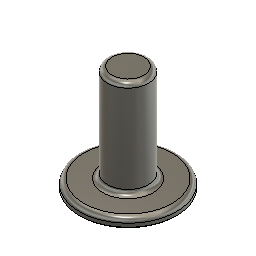
Stick_Topper (Autodesk Fusion 360 archive; units mm, degrees)
design "Stick Topper"
part number: Medium
Autodesk Fusion 360 part; units mm, degrees
sketch "Sketch1" plane through (0, 0, 0) normal (0, 0, 1) x (1, 0, 0)
  line L0 (0, 0) -> (14, 0)
  line L1 (14, 0) -> (14, -6)
  line L2 (14, -6) -> (41.5, -6)
  line L3 (41.5, -6) -> (41.5, 2)
  line L4 (41.5, 2) -> (17.5, 2)
  line L5 (17.5, 2) -> (17.5, 85)
  line L6 (17.5, 85) -> (0, 85)
  line L7 (0, 85) -> (0, 0)
  line L8 (9, 0) -> (7.6706, 3)
  line L9 (7.6706, 3) -> (0, 3)
  line L10 (14.995, 4) -> (14.995, 82)
  line L11 (14.995, 82) -> (0, 82)
  line L12 (14.995, 4) -> (0, 4)
  dimension "d1" = 2
  dimension "d3" = 85
  dimension "d4" = 17.5
  dimension "d5" = 6
  dimension "d6" = 14
  dimension "d10" = 3
  dimension "d11" = 66.1
  dimension "d12" = 9
  dimension "d22" = 3
  dimension "d24" = 24
  dimension "d27" = 2.505
  dimension "d28" = 1
  constraint coincident L0.start L7.end
  constraint horizontal L0
  constraint perpendicular L0 L1
  constraint perpendicular L1 L2
  constraint perpendicular L0 L3
  constraint perpendicular L3 L4
  constraint perpendicular L0 L5
  constraint perpendicular L6 L7
  constraint coincident L0 L8.start
  constraint coincident L7 L9.end
  constraint perpendicular L7 L9
  constraint coincident L7 L11.end
  constraint perpendicular L7 L11
  constraint perpendicular L9 L10
  constraint coincident L8.end L9.start
  constraint coincident L7 L12.end
  constraint perpendicular L7 L12
  measures "d1" distance of L0 L4
  measures "d3" distance of L6.end L0.start
  measures "d4" distance of L5.end L6.end
  measures "d5" distance of L0.end L1.end
  measures "d6" distance of L0.start L0.end
  measures "d10" distance of L0 L9
  measures "d11" angle of L0 L8
  measures "d12" distance of L0.start L8.start
  measures "d22" distance of L6 L11
  measures "d24" distance of L3 L5
  measures "d27" distance of L5 L10
  measures "d28" distance of L9 L12
revolve "Revolve1" add sketch "Sketch1" angle 360 about axis through (0, 85, 0) along (0, -1, 0) contours L0 L1 L2 L3 L4 L5 L6 L7 L8 L9 L10 L11 L12
fillet "Fillet1" radius 4 2 edges at (-16.3157, 2, -6.3283) (-38.6916, 2, -15.007)
fillet "Fillet1" radius 4 1 edges at (-16.3157, 85, -6.3283)
thread "Thread1" "ISO Metric profile 28.0 M28x2 6H" major diameter 28.2565 minor diameter 26.0224 pitch 2 angle 60 modelled right hand crest width 0.5434 on face at (13.9304, -4, -1.3939) crest through (13.0112, -0.5, 0)
chamfer "Chamfer1" distance 1 angle 45 1 edges at (-38.6916, -6, -15.007)
sketch "Sketch2" plane through (0, 0, 0) normal (0, -1, 0) x (1, 0, 0)
  arc A0 (-9.8061, -8.5517) -> (9.8061, -8.5517) centre (0, 0) ccw
  spline S0 degree 3 poles (9.8061, -8.5517) (10.5142, -7.806) (11.1313, -6.9789) (12.1649, -5.1889) (12.5756, -4.2311) (13.3644, -1.5664) (13.5251, 0.1832) (13.1691, 3.6743) (12.6452, 5.381) (10.964, 8.5248) (9.8136, 9.9266) (7.0217, 12.2323) (5.4004, 13.1058) (3.6576, 13.6466) knots -2.761439 -2.761439 -2.761439 -2.761439 -2.452475 -2.452475 -2.140473 -2.140473 -1.617666 -1.617666 -1.08665 -1.08665 -0.547427 -0.547427 0 0 0 0
  arc A1 (3.6576, 13.6466) -> (-3.6576, 13.6466) centre (0, 0) ccw
  spline S1 degree 3 poles (-3.6576, 13.6466) (-4.7143, 13.3187) (-5.7287, 12.8678) (-7.6214, 11.7415) (-8.4942, 11.0722) (-10.5613, 9.057) (-11.589, 7.5703) (-13.0011, 4.3098) (-13.3814, 2.5718) (-13.4489, -0.9248) (-13.1459, -2.6494) (-11.901, -5.8577) (-10.9811, -7.3143) (-9.8061, -8.5517) knots -2.756672 -2.756672 -2.756672 -2.756672 -2.425266 -2.425266 -2.096892 -2.096892 -1.560377 -1.560377 -1.032054 -1.032054 -0.511928 -0.511928 0 0 0 0
  circle A2 centre (0, 0) radius 40.5
  line L0 (-39.4873, 9) -> (39.4873, 9)
  line L1 (9, 39.4873) -> (9, -39.4873)
  line L2 (39.4873, -9) -> (-39.4873, -9)
  line L3 (-9, -39.4873) -> (-9, 39.4873)
  circle A3 centre (0, 0) radius 9
  constraint coincident A2 L0.start
  constraint coincident A2 L0.end
  constraint horizontal L0
  constraint coincident A2 L1.start
  constraint coincident A2 L1.end
  constraint perpendicular L0 L1
  constraint coincident A2 L2.start
  constraint coincident A2 L2.end
  constraint perpendicular L1 L2
  constraint coincident A2 L3.start
  constraint coincident A2 L3.end
  constraint perpendicular L2 L3
  constraint tangent L2 A3
  constraint tangent L3 A3
  constraint tangent L0 A3
  constraint tangent L1 A3
extrude "Extrude1" cut sketch "Sketch2" against normal blind 0.4 contours L2 L3 A3 | L0 L3 A3 | L1 L2 A3 | A3 | L0 L1 A3
extrude "Extrude2" cut sketch "Sketch2" against normal blind 0.2 contours A0 L1 L2 L3 | S0 A1 S1 L0 L1 L3
chamfer "Chamfer2" distance 2 angle 45 1 edges at (-13.9802, 82, -5.4224)
chamfer "Chamfer3" distance 0.4 angle 45 1 edges at (-8.2257, 0.4, -3.1904)
fillet "Fillet2" radius 2 1 edges at (-13.9802, 4, -5.4224)
equation "d3 = Height"
equation "d4 = Diameter / 2"
equation "Height = 85 mm" comment "Minimum 9mm"
equation "Diameter = 35 mm" comment "Minumum 9mm"
equation "d24 = Base_Brim + 4 mm"
equation "Base_Brim = 20 mm" comment "Model adds 4mm to input"
equation "d27 = ( 1.67 * 1.5 ) * 1 mm"
named bodies: "Stick_Topper"
